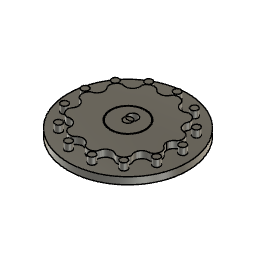
Example Result v0 (Autodesk Fusion 360 design; units mm, degrees)
Autodesk Fusion 360 part; units mm, degrees
sketch "diskSketch" plane through (0, 0, 0) normal (0, 0, 1) x (1, 0, 0)
  spline S0 degree 5 number of poles 1805
  spline S1 degree 5 number of poles 1805
  spline S2 degree 3 poles (27.5, 0) (27.5, -0.8364) (27.7298, -1.6288) (27.9895, -2.1783) (28.3571, -2.9563) (28.7204, -3.3302) (28.9647, -3.582) (29.3501, -3.9791) (29.5444, -4.104) (29.6826, -4.2063) (29.9351, -4.3932) (29.9974, -4.4285) (30.0646, -4.475) (30.2296, -4.589) (30.2633, -4.6167) (30.3364, -4.6819) (30.5367, -4.8606) (30.8163, -5.1989) (31.0395, -5.7169) (31.3799, -6.5067) (31.5244, -7.6667) (31.2804, -8.7782) (31.0439, -9.8558) (30.4517, -10.869) (29.7612, -11.5227) (29.2524, -12.0044) (28.7053, -12.2856) (28.3272, -12.3989) (28.1828, -12.4422) (28.0593, -12.4636) (27.9596, -12.4749) (27.9048, -12.4811) (27.8974, -12.4821) (27.7486, -12.4878) (27.6622, -12.4911) (27.5665, -12.4944) (27.4556, -12.4988) (27.3788, -12.5019) (27.2857, -12.4897) (26.842, -12.5475) (26.5223, -12.5891) (26.0046, -12.6545) (25.2479, -13.0138) (24.7458, -13.2522) (24.1194, -13.646) (23.5495, -14.3118) (23.0297, -14.919) (22.6138, -15.7656) (22.4459, -16.5212) (22.2613, -17.3526) (22.3204, -18.0094) (22.386, -18.4313) (22.4877, -19.0857) (22.5909, -19.29) (22.642, -19.4348) (22.7121, -19.6333) (22.7474, -19.717) (22.7899, -19.8212) (22.8708, -20.0199) (22.9081, -20.104) (22.9231, -20.142) (22.9596, -20.2349) (22.9966, -20.3483) (23.0229, -20.4798) (23.0861, -20.796) (23.1033, -21.3457) (22.941, -21.9659) (22.7031, -22.875) (22.0726, -23.9098) (21.187, -24.6432) (20.3584, -25.3292) (19.3241, -25.7421) (18.4538, -25.8362) (17.8604, -25.9004) (17.353, -25.8209) (17.045, -25.7203) (16.9404, -25.6861) (16.8631, -25.6529) (16.7756, -25.6098) (16.723, -25.584) (16.7225, -25.5844) (16.6515, -25.5425) (16.6091, -25.5175) (16.5151, -25.4606) (16.4071, -25.3973) (16.3212, -25.347) (16.2748, -25.3194) (16.1409, -25.2452) (16.052, -25.196) (15.9195, -25.1081) (15.5103, -24.9416) (15.1789, -24.8066) (14.6328, -24.6047) (13.8187, -24.5618) (13.0612, -24.5218) (12.0837, -24.6809) (11.2521, -25.0993) (10.3608, -25.5476) (9.6892, -26.2416) (9.296, -26.8297) (8.8257, -27.5333) (8.6839, -28.0536) (8.6021, -28.3468) (8.482, -28.7769) (8.489, -28.8266) (8.4745, -28.9021) (8.4406, -29.0782) (8.4026, -29.2946) (8.392, -29.3494) (8.3809, -29.4064) (8.3746, -29.4314) (8.3564, -29.4951) (8.316, -29.6367) (8.2697, -29.7576) (8.1789, -29.9291) (7.9347, -30.3903) (7.4012, -31.0102) (6.6342, -31.4665) (5.714, -32.014) (4.4821, -32.3033) (3.3558, -32.2059) (2.3425, -32.1183) (1.4347, -31.7209) (0.8897, -31.2936) (0.6133, -31.0769) (0.4328, -30.8653) (0.3291, -30.7121) (0.2863, -30.6489) (0.2436, -30.5766) (0.2081, -30.5089) (0.1823, -30.4595) (0.1408, -30.3648) (-0.0014, -30.0921) (-0.0541, -29.991) (-0.1025, -29.8918) (-0.2461, -29.6587) (-0.3423, -29.5025) (-0.4742, -29.2688) (-0.8391, -28.8643) (-1.1195, -28.5534) (-1.5694, -28.1164) (-2.2864, -27.7436) (-2.9439, -27.4017) (-3.8232, -27.1741) (-4.6043, -27.1692) (-5.4948, -27.1637) (-6.1979, -27.3848) (-6.6882, -27.5989) (-7.4716, -27.941) (-7.8317, -28.2711) (-8.0745, -28.4848) (-8.476, -28.8382) (-8.5172, -28.9164) (-8.5762, -28.9799) (-8.7072, -29.1206) (-8.8019, -29.2219) (-8.8412, -29.2609) (-8.912, -29.3312) (-9.005, -29.4114) (-9.1302, -29.4954) (-9.5088, -29.7495) (-10.2824, -30.0502) (-11.2002, -30.0607) (-12.294, -30.0733) (-13.5598, -29.6739) (-14.5105, -28.9669) (-15.3604, -28.3349) (-15.9413, -27.4715) (-16.1735, -26.797) (-16.2958, -26.442) (-16.3282, -26.1649) (-16.328, -25.9607) (-16.3279, -25.8747) (-16.3261, -25.8385) (-16.3063, -25.6536) (-16.2985, -25.5807) (-16.2912, -25.5258) (-16.2741, -25.3561) (-16.2616, -25.2314) (-16.2255, -25.0355) (-16.2432, -24.5221) (-16.2531, -24.2338) (-16.2694, -23.8438) (-16.4483, -23.2265) (-16.5847, -22.7558) (-16.8375, -22.1165) (-17.3604, -21.4595) (-17.8554, -20.8375) (-18.6109, -20.2666) (-19.3143, -19.9609) (-20.0832, -19.6267) (-20.7177, -19.5586) (-21.1477, -19.5403) (-21.8219, -19.5117) (-22.1004, -19.5816) (-22.307, -19.6171) (-22.6555, -19.6769) (-22.7856, -19.7171) (-22.8998, -19.7464) (-23.1587, -19.8128) (-23.1843, -19.8205) (-23.2501, -19.8343) (-23.4304, -19.8721) (-23.6097, -19.8913) (-23.8896, -19.8684) (-24.4796, -19.8201) (-25.3885, -19.5117) (-26.1748, -18.8757) (-27.0038, -18.2052) (-27.6841, -17.1908) (-27.9911, -16.1567) (-28.2675, -15.2257) (-28.235, -14.2921) (-28.0634, -13.6842) (-27.9892, -13.4213) (-27.9, -13.2271) (-27.815, -13.083) (-27.7771, -13.0188) (-27.7302, -12.9492) (-27.7028, -12.9124) (-27.6844, -12.8876) (-27.6489, -12.8431) (-27.5569, -12.7286) (-27.5038, -12.6625) (-27.4564, -12.6033) (-27.4033, -12.5363) (-27.3615, -12.4835) (-27.3087, -12.4318) (-27.1123, -12.1457) (-26.9522, -11.9125) (-26.6641, -11.5059) (-26.4205, -10.734) (-26.2398, -10.1613) (-26.1008, -9.3649) (-26.235, -8.4458) (-26.3558, -7.6193) (-26.739, -6.7287) (-27.2269, -6.0891) (-27.7439, -5.4112) (-28.294, -5.0252) (-28.665, -4.8012) (-29.2451, -4.451) (-29.4567, -4.4063) (-29.5843, -4.358) (-29.7507, -4.2949) (-29.8157, -4.2735) (-29.9166, -4.2392) (-30.0953, -4.1785) (-30.2009, -4.1453) (-30.2363, -4.133) (-30.2851, -4.116) (-30.3346, -4.0961) (-30.3964, -4.0682) (-30.5109, -4.0166) (-30.6072, -3.9633) (-30.742, -3.8694) (-31.1329, -3.5971) (-31.6402, -3.0544) (-31.9935, -2.3069) (-32.4399, -1.3624) (-32.6142, -0.118) (-32.4095, 1.0026) (-32.2576, 1.8342) (-31.9068, 2.5902) (-31.499, 3.1259) (-31.2419, 3.4636) (-30.9701, 3.711) (-30.7392, 3.8713) (-30.5825, 3.9801) (-30.4714, 4.0378) (-30.3366, 4.0942) (-30.2813, 4.1173) (-30.2756, 4.1201) (-30.1976, 4.1462) (-30.1459, 4.1634) (-30.0203, 4.2035) (-29.8763, 4.253) (-29.7877, 4.2834) (-29.728, 4.3034) (-29.5798, 4.3597) (-29.46, 4.4052) (-29.2683, 4.4545) (-28.7732, 4.7376) (-28.4321, 4.9327) (-27.9182, 5.2633) (-27.3929, 5.8827) (-26.9035, 6.4599) (-26.4683, 7.2978) (-26.293, 8.1223) (-26.0881, 9.0859) (-26.1992, 9.9611) (-26.3764, 10.5866) (-26.6142, 11.4261) (-26.925, 11.87) (-27.096, 12.1219) (-27.3408, 12.4823) (-27.3781, 12.5046) (-27.424, 12.5623) (-27.515, 12.6769) (-27.6332, 12.8228) (-27.6725, 12.8729) (-27.7163, 12.9287) (-27.7233, 12.9391) (-27.7575, 12.9911) (-27.8417, 13.1187) (-27.9123, 13.25) (-27.9871, 13.4502) (-28.1807, 13.9688) (-28.2892, 14.8359) (-28.0932, 15.7558) (-27.8673, 16.8165) (-27.2406, 17.9172) (-26.412, 18.672) (-25.665, 19.3525) (-24.769, 19.7379) (-24.1169, 19.841) (-23.7892, 19.8928) (-23.5487, 19.8831) (-23.3653, 19.8552) (-23.3028, 19.8457) (-23.2472, 19.8348) (-23.1696, 19.816) (-23.1079, 19.801) (-23.0329, 19.7773) (-22.7561, 19.7106) (-22.6382, 19.6821) (-22.5014, 19.6455) (-22.1939, 19.5988) (-21.9926, 19.5682) (-21.7155, 19.5183) (-21.1676, 19.5395) (-20.7578, 19.5554) (-20.1633, 19.6148) (-19.4304, 19.9121) (-18.7619, 20.1833) (-18.0201, 20.6943) (-17.5047, 21.2862) (-16.9391, 21.9357) (-16.6447, 22.6034) (-16.4874, 23.0977) (-16.2407, 23.8734) (-16.2454, 24.3147) (-16.2406, 24.6279) (-16.232, 25.1873) (-16.2715, 25.3348) (-16.2831, 25.442) (-16.3005, 25.6029) (-16.3098, 25.6825) (-16.3165, 25.753) (-16.3288, 25.8813) (-16.3292, 25.9161) (-16.3276, 26.0013) (-16.3228, 26.2464) (-16.2669, 26.5994) (-16.0832, 27.0318) (-15.7711, 27.7665) (-15.0765, 28.6349) (-14.1404, 29.2194) (-13.1966, 29.8087) (-12.0276, 30.1013) (-11.0333, 30.056) (-10.3394, 30.0243) (-9.7408, 29.8356) (-9.3544, 29.6294) (-9.1559, 29.5235) (-9.0203, 29.4228) (-8.912, 29.3271) (-8.8658, 29.2862) (-8.8531, 29.2748) (-8.7838, 29.202) (-8.7349, 29.1507) (-8.6604, 29.0703) (-8.5751, 28.9786) (-8.5254, 28.9252) (-8.4787, 28.8629) (-8.2345, 28.6311) (-8.049, 28.4551) (-7.7634, 28.1655) (-7.1134, 27.8081) (-6.7184, 27.5909) (-6.1661, 27.3374) (-5.3667, 27.2217) (-4.6642, 27.1201) (-3.7569, 27.1776) (-2.9737, 27.4481) (-2.162, 27.7285) (-1.5452, 28.1805) (-1.1609, 28.5377) (-0.598, 29.0607) (-0.4197, 29.3848) (-0.2935, 29.5829) (-0.1127, 29.8668) (-0.066, 29.9688) (-0.0091, 30.0774) (0.2217, 30.5179) (0.2057, 30.5088) (0.2538, 30.5917) (0.3361, 30.7335) (0.4253, 30.8582) (0.5862, 31.0229) (0.9753, 31.4213) (1.7542, 31.9081) (2.7129, 32.1108) (3.7766, 32.3358) (5.0356, 32.2101) (6.0583, 31.7621) (6.7284, 31.4686) (7.2951, 31.0465) (7.6822, 30.6225) (7.9524, 30.3264) (8.1342, 30.0354) (8.243, 29.7997) (8.3005, 29.6752) (8.3306, 29.5884) (8.3609, 29.4793) (8.3778, 29.4183) (8.3814, 29.4047) (8.3938, 29.3399) (8.403, 29.2915) (8.4292, 29.1419) (8.455, 29.0044) (8.47, 28.9245) (8.474, 28.8947) (8.5108, 28.721) (8.5373, 28.5959) (8.5681, 28.3644) (8.7663, 27.8511) (8.9305, 27.426) (9.2319, 26.7809) (9.8645, 26.1231) (10.415, 25.5505) (11.2404, 25.0128) (12.1257, 24.7564) (13.026, 24.4956) (13.9153, 24.5301) (14.5283, 24.6489) (15.3068, 24.7998) (15.6828, 25.01) (15.8931, 25.1147) (16.1845, 25.2599) (16.2151, 25.2865) (16.285, 25.3266) (16.4234, 25.406) (16.5925, 25.5077) (16.6517, 25.5426) (16.7242, 25.5854) (16.7249, 25.5851) (16.7795, 25.6118) (16.9246, 25.6828) (17.0645, 25.7361) (17.2801, 25.7845) (17.7791, 25.8965) (18.5768, 25.8984) (19.4027, 25.631) (20.4105, 25.3047) (21.4331, 24.5804) (22.1043, 23.6778) (22.6277, 22.9741) (22.9366, 22.1737) (23.0328, 21.5172) (23.1018, 21.0463) (23.0627, 20.6449) (23.0093, 20.4173) (22.9887, 20.3292) (22.9554, 20.2264) (22.93, 20.1597) (22.9153, 20.1214) (22.8933, 20.0721) (22.8111, 19.873) (22.7704, 19.7744) (22.7302, 19.6763) (22.672, 19.518) (22.6324, 19.4102) (22.572, 19.2776) (22.4727, 18.8679) (22.3989, 18.5631) (22.2832, 18.0707) (22.3357, 17.2884) (22.3779, 16.6599) (22.5777, 15.8389) (22.9826, 15.1214) (23.4111, 14.362) (24.0166, 13.779) (24.5504, 13.4143) (25.3758, 12.8504) (26.0286, 12.6983) (26.4611, 12.6107) (27.123, 12.4766) (27.3047, 12.5052) (27.4079, 12.5008) (27.5295, 12.4956) (27.5867, 12.4938) (27.6726, 12.4906) (27.8267, 12.4849) (27.8822, 12.4822) (27.9215, 12.4787) (27.9981, 12.472) (28.125, 12.4535) (28.2503, 12.4206) (28.6521, 12.315) (29.3279, 11.9787) (29.9133, 11.372) (30.6239, 10.6357) (31.1877, 9.5184) (31.3523, 8.383) (31.5133, 7.2733) (31.2858, 6.169) (30.9215, 5.4678) (30.7394, 5.1172) (30.5374, 4.8717) (30.3815, 4.7234) (30.3035, 4.6493) (30.2602, 4.6127) (30.1351, 4.5242) (30.0815, 4.4862) (30.0264, 4.4499) (29.8663, 4.3382) (29.7692, 4.2704) (29.6334, 4.1879) (29.3172, 3.9145) (29.1277, 3.7506) (28.8612, 3.5354) (28.4682, 2.9898) (28.2075, 2.6278) (27.8772, 2.0856) (27.67, 1.3043) (27.565, 0.9081) (27.5, 0.4556) (27.5, 0) knots 0 0 0 0 0.0004895 0.0004895 0.0004895 0.00118259 0.00118259 0.00118259 0.00227595 0.00227595 0.00227595 0.00427422 0.00427422 0.00427422 0.00917873 0.00917873 0.00917873 0.02262065 0.02262065 0.02262065 0.04311537 0.04311537 0.04311537 0.0629846 0.0629846 0.0629846 0.07762546 0.07762546 0.07762546 0.08321474 0.08321474 0.08321474 0.08628579 0.08628579 0.08628579 0.08807039 0.08807039 0.08807039 0.08930494 0.08930494 0.08930494 0.09019429 0.09019429 0.09019429 0.09078445 0.09078445 0.09078445 0.09132266 0.09132266 0.09132266 0.09191484 0.09191484 0.09191484 0.09283321 0.09283321 0.09283321 0.09409235 0.09409235 0.09409235 0.09649245 0.09649245 0.09649245 0.10235615 0.10235615 0.10235615 0.11645429 0.11645429 0.11645429 0.13711768 0.13711768 0.13711768 0.15644901 0.15644901 0.15644901 0.1696295 0.1696295 0.1696295 0.1741071 0.1741071 0.1741071 0.17679588 0.17679588 0.17679588 0.1784037 0.1784037 0.1784037 0.17968093 0.17968093 0.17968093 0.18052857 0.18052857 0.18052857 0.18121516 0.18121516 0.18121516 0.18185402 0.18185402 0.18185402 0.18253869 0.18253869 0.18253869 0.18335769 0.18335769 0.18335769 0.18455897 0.18455897 0.18455897 0.18735939 0.18735939 0.18735939 0.19026496 0.19026496 0.19026496 0.19672698 0.19672698 0.19672698 0.21410686 0.21410686 0.21410686 0.2349604 0.2349604 0.2349604 0.25372072 0.25372072 0.25372072 0.26323468 0.26323468 0.26323468 0.26716265 0.26716265 0.26716265 0.2700253 0.2700253 0.2700253 0.27108749 0.27108749 0.27108749 0.27179932 0.27179932 0.27179932 0.27234648 0.27234648 0.27234648 0.27284827 0.27284827 0.27284827 0.2734204 0.2734204 0.2734204 0.27433454 0.27433454 0.27433454 0.27584592 0.27584592 0.27584592 0.27920032 0.27920032 0.27920032 0.28524135 0.28524135 0.28524135 0.30350219 0.30350219 0.30350219 0.32526775 0.32526775 0.32526775 0.344725 0.344725 0.344725 0.35496367 0.35496367 0.35496367 0.35927589 0.35927589 0.35927589 0.36097586 0.36097586 0.36097586 0.36222396 0.36222396 0.36222396 0.36292478 0.36292478 0.36292478 0.36345931 0.36345931 0.36345931 0.36396532 0.36396532 0.36396532 0.36451839 0.36451839 0.36451839 0.3653857 0.3653857 0.3653857 0.36684904 0.36684904 0.36684904 0.37016576 0.37016576 0.37016576 0.37924482 0.37924482 0.37924482 0.39838777 0.39838777 0.39838777 0.41856891 0.41856891 0.41856891 0.43673863 0.43673863 0.43673863 0.44459901 0.44459901 0.44459901 0.44809961 0.44809961 0.44809961 0.4504535 0.4504535 0.4504535 0.45181271 0.45181271 0.45181271 0.45288339 0.45288339 0.45288339 0.45375646 0.45375646 0.45375646 0.4544043 0.4544043 0.4544043 0.45498694 0.45498694 0.45498694 0.45560434 0.45560434 0.45560434 0.45656983 0.45656983 0.45656983 0.45782948 0.45782948 0.45782948 0.46005992 0.46005992 0.46005992 0.46312902 0.46312902 0.46312902 0.46880455 0.46880455 0.46880455 0.48526725 0.48526725 0.48526725 0.5060698 0.5060698 0.5060698 0.52150512 0.52150512 0.52150512 0.53123486 0.53123486 0.53123486 0.53783732 0.53783732 0.53783732 0.54054314 0.54054314 0.54054314 0.54233789 0.54233789 0.54233789 0.5434415 0.5434415 0.5434415 0.54433321 0.54433321 0.54433321 0.54494776 0.54494776 0.54494776 0.54552032 0.54552032 0.54552032 0.54618951 0.54618951 0.54618951 0.54708756 0.54708756 0.54708756 0.54837287 0.54837287 0.54837287 0.55092383 0.55092383 0.55092383 0.55376597 0.55376597 0.55376597 0.56074285 0.56074285 0.56074285 0.57881743 0.57881743 0.57881743 0.59965766 0.59965766 0.59965766 0.61844581 0.61844581 0.61844581 0.62788938 0.62788938 0.62788938 0.63111017 0.63111017 0.63111017 0.63366994 0.63366994 0.63366994 0.63475964 0.63475964 0.63475964 0.635473 0.635473 0.635473 0.63600667 0.63600667 0.63600667 0.63649349 0.63649349 0.63649349 0.63702765 0.63702765 0.63702765 0.63786593 0.63786593 0.63786593 0.63936372 0.63936372 0.63936372 0.64160996 0.64160996 0.64160996 0.64569763 0.64569763 0.64569763 0.65746357 0.65746357 0.65746357 0.67745587 0.67745587 0.67745587 0.69761487 0.69761487 0.69761487 0.7116825 0.7116825 0.7116825 0.71890829 0.71890829 0.71890829 0.72199175 0.72199175 0.72199175 0.72416369 0.72416369 0.72416369 0.72543114 0.72543114 0.72543114 0.72639376 0.72639376 0.72639376 0.72697867 0.72697867 0.72697867 0.72749264 0.72749264 0.72749264 0.72802538 0.72802538 0.72802538 0.7288056 0.7288056 0.7288056 0.72992363 0.72992363 0.72992363 0.73445822 0.73445822 0.73445822 0.74221478 0.74221478 0.74221478 0.76097264 0.76097264 0.76097264 0.78178556 0.78178556 0.78178556 0.79542396 0.79542396 0.79542396 0.80494586 0.80494586 0.80494586 0.80997549 0.80997549 0.80997549 0.81279025 0.81279025 0.81279025 0.81489378 0.81489378 0.81489378 0.81611582 0.81611582 0.81611582 0.81699629 0.81699629 0.81699629 0.81772554 0.81772554 0.81772554 0.81836023 0.81836023 0.81836023 0.81900578 0.81900578 0.81900578 0.81982558 0.81982558 0.81982558 0.82096133 0.82096133 0.82096133 0.8232058 0.8232058 0.8232058 0.8259593 0.8259593 0.8259593 0.83328439 0.83328439 0.83328439 0.85024081 0.85024081 0.85024081 0.87093352 0.87093352 0.87093352 0.88706683 0.88706683 0.88706683 0.89863825 0.89863825 0.89863825 0.90311813 0.90311813 0.90311813 0.9056923 0.9056923 0.9056923 0.90696765 0.90696765 0.90696765 0.90783657 0.90783657 0.90783657 0.90848293 0.90848293 0.90848293 0.90900219 0.90900219 0.90900219 0.90955175 0.90955175 0.90955175 0.9104014 0.9104014 0.9104014 0.91170187 0.91170187 0.91170187 0.91323489 0.91323489 0.91323489 0.91598534 0.91598534 0.91598534 0.92133468 0.92133468 0.92133468 0.9384865 0.9384865 0.9384865 0.95930437 0.95930437 0.95930437 0.97965218 0.97965218 0.97965218 0.98982609 0.98982609 0.98982609 0.99491305 0.99491305 0.99491305 0.99709279 0.99709279 0.99709279 0.99841498 0.99841498 0.99841498 0.99920749 0.99920749 0.99920749 0.99973334 0.99973334 0.99973334 1 1 1 1
  circle A0 centre (0, 0) radius 12.5
  point P0 (32.5492, -0.096)
  point P1 (32.6945, -0.2144)
  point P2 (32.9288, -0.3765)
  point P3 (33.2407, -0.6017)
  point P4 (33.615, -0.9067)
  point P5 (34.0333, -1.3046)
  point P6 (34.4748, -1.8043)
  point P7 (34.9171, -2.4105)
  point P8 (35.3377, -3.123)
  point P9 (35.7141, -3.9367)
  point P10 (36.0256, -4.8423)
  point P11 (36.2537, -5.8263)
  point P12 (36.3833, -6.8717)
  point P13 (36.403, -7.9585)
  point P14 (36.3057, -9.0651)
  point P15 (36.089, -10.1688)
  point P16 (35.7555, -11.2468)
  point P17 (35.312, -12.2774)
  point P18 (34.7701, -13.2409)
  point P19 (34.145, -14.1201)
  point P20 (33.4551, -14.9017)
  point P21 (32.7214, -15.5763)
  point P22 (31.9661, -16.139)
  point P23 (31.2121, -16.5898)
  point P24 (30.4818, -16.9332)
  point P25 (29.796, -17.1783)
  point P26 (29.1733, -17.3384)
  point P27 (28.629, -17.4302)
  point P28 (28.1747, -17.4731)
  point P29 (27.8174, -17.4887)
  point P30 (27.5599, -17.4993)
  point P31 (27.3998, -17.5272)
  point P32 (27.3302, -17.5941)
  point P33 (27.34, -17.7191)
  point P34 (27.414, -17.9192)
  point P35 (27.534, -18.2073)
  point P36 (27.6794, -18.5925)
  point P37 (27.8281, -19.0793)
  point P38 (27.9574, -19.6675)
  point P39 (28.0451, -20.3522)
  point P40 (28.0706, -21.1239)
  point P41 (28.0156, -21.9691)
  point P42 (27.865, -22.8706)
  point P43 (27.6073, -23.8088)
  point P44 (27.2358, -24.7617)
  point P45 (26.748, -25.7068)
  point P46 (26.1464, -26.6211)
  point P47 (25.4381, -27.4831)
  point P48 (24.6346, -28.273)
  point P49 (23.751, -28.9737)
  point P50 (22.806, -29.5719)
  point P51 (21.8203, -30.0582)
  point P52 (20.8164, -30.4279)
  point P53 (19.817, -30.6809)
  point P54 (18.8445, -30.8219)
  point P55 (17.9199, -30.8601)
  point P56 (17.0617, -30.8088)
  point P57 (16.2852, -30.6849)
  point P58 (15.6021, -30.508)
  point P59 (15.0196, -30.2996)
  point P60 (14.5402, -30.0824)
  point P61 (14.1619, -29.8788)
  point P62 (13.8777, -29.7104)
  point P63 (13.6766, -29.5968)
  point P64 (13.5437, -29.5547)
  point P65 (13.4607, -29.5976)
  point P66 (13.4072, -29.7344)
  point P67 (13.3612, -29.9697)
  point P68 (13.3001, -30.3036)
  point P69 (13.2019, -30.7311)
  point P70 (13.0461, -31.2428)
  point P71 (12.8146, -31.8252)
  point P72 (12.4922, -32.4615)
  point P73 (12.0677, -33.1316)
  point P74 (11.5344, -33.814)
  point P75 (10.89, -34.4858)
  point P76 (10.137, -35.1245)
  point P77 (9.2825, -35.7083)
  point P78 (8.338, -36.2174)
  point P79 (7.319, -36.6349)
  point P80 (6.2437, -36.9474)
  point P81 (5.1333, -37.1456)
  point P82 (4.0099, -37.2247)
  point P83 (2.8964, -37.1848)
  point P84 (1.8153, -37.0306)
  point P85 (0.7873, -36.7713)
  point P86 (-0.169, -36.4204)
  point P87 (-1.0383, -35.9947)
  point P88 (-1.809, -35.5141)
  point P89 (-2.474, -35.0001)
  point P90 (-3.0306, -34.4754)
  point P91 (-3.4812, -33.9627)
  point P92 (-3.8324, -33.4838)
  point P93 (-4.0956, -33.0582)
  point P94 (-4.2855, -32.7031)
  point P95 (-4.4205, -32.4317)
  point P96 (-4.5209, -32.2535)
  point P97 (-4.6088, -32.1732)
  point P98 (-4.7067, -32.1908)
  point P99 (-4.8365, -32.3017)
  point P100 (-5.0187, -32.4965)
  point P101 (-5.2715, -32.7621)
  point P102 (-5.6098, -33.0815)
  point P103 (-6.0447, -33.4349)
  point P104 (-6.583, -33.8009)
  point P105 (-7.2269, -34.1568)
  point P106 (-7.9739, -34.48)
  point P107 (-8.8166, -34.7489)
  point P108 (-9.7436, -34.9437)
  point P109 (-10.7394, -35.0475)
  point P110 (-11.7856, -35.0471)
  point P111 (-12.8612, -34.9332)
  point P112 (-13.9439, -34.701)
  point P113 (-15.0108, -34.3506)
  point P114 (-16.0396, -33.8868)
  point P115 (-17.0094, -33.3188)
  point P116 (-17.9017, -32.66)
  point P117 (-18.7013, -31.9275)
  point P118 (-19.3966, -31.141)
  point P119 (-19.9805, -30.3222)
  point P120 (-20.4507, -29.4938)
  point P121 (-20.8092, -28.6786)
  point P122 (-21.0631, -27.8982)
  point P123 (-21.2236, -27.1727)
  point P124 (-21.3058, -26.5189)
  point P125 (-21.328, -25.9504)
  point P126 (-21.3106, -25.4767)
  point P127 (-21.2759, -25.1026)
  point P128 (-21.2464, -24.8284)
  point P129 (-21.2441, -24.6494)
  point P130 (-21.2896, -24.5567)
  point P131 (-21.4011, -24.537)
  point P132 (-21.5936, -24.5736)
  point P133 (-21.8782, -24.647)
  point P134 (-22.2618, -24.7357)
  point P135 (-22.7466, -24.8173)
  point P136 (-23.3299, -24.8693)
  point P137 (-24.0046, -24.8701)
  point P138 (-24.7591, -24.8003)
  point P139 (-25.5781, -24.643)
  point P140 (-26.4429, -24.385)
  point P141 (-27.3327, -24.0171)
  point P142 (-28.225, -23.5347)
  point P143 (-29.0971, -22.9378)
  point P144 (-29.9266, -22.2313)
  point P145 (-30.6927, -21.4244)
  point P146 (-31.3768, -20.5307)
  point P147 (-31.9636, -19.5671)
  point P148 (-32.4419, -18.5533)
  point P149 (-32.8044, -17.5112)
  point P150 (-33.0488, -16.4635)
  point P151 (-33.1775, -15.4327)
  point P152 (-33.1973, -14.4409)
  point P153 (-33.1197, -13.5076)
  point P154 (-32.9599, -12.6501)
  point P155 (-32.7362, -11.8818)
  point P156 (-32.4693, -11.2123)
  point P157 (-32.1815, -10.6463)
  point P158 (-31.8955, -10.1842)
  point P159 (-31.6335, -9.8214)
  point P160 (-31.4162, -9.549)
  point P161 (-31.2619, -9.3538)
  point P162 (-31.1859, -9.2192)
  point P163 (-31.1993, -9.1258)
  point P164 (-31.3092, -9.0521)
  point P165 (-31.5178, -8.9759)
  point P166 (-31.8227, -8.8748)
  point P167 (-32.2167, -8.7274)
  point P168 (-32.6884, -8.5142)
  point P169 (-33.2226, -8.2186)
  point P170 (-33.8006, -7.8274)
  point P171 (-34.4017, -7.3316)
  point P172 (-35.0036, -6.7266)
  point P173 (-35.5833, -6.0125)
  point P174 (-36.1187, -5.1943)
  point P175 (-36.5889, -4.2814)
  point P176 (-36.9753, -3.2871)
  point P177 (-37.2629, -2.2286)
  point P178 (-37.4401, -1.1257)
  point P179 (-37.5, 0)
  point P180 (-37.4401, 1.1257)
  point P181 (-37.2629, 2.2286)
  point P182 (-36.9753, 3.2871)
  point P183 (-36.5889, 4.2814)
  point P184 (-36.1187, 5.1943)
  point P185 (-35.5833, 6.0125)
  point P186 (-35.0036, 6.7266)
  point P187 (-34.4017, 7.3316)
  point P188 (-33.8006, 7.8274)
  point P189 (-33.2226, 8.2186)
  point P190 (-32.6884, 8.5142)
  point P191 (-32.2167, 8.7274)
  point P192 (-31.8227, 8.8748)
  point P193 (-31.5178, 8.9759)
  point P194 (-31.3092, 9.0521)
  point P195 (-31.1993, 9.1258)
  point P196 (-31.1859, 9.2192)
  point P197 (-31.2619, 9.3538)
  point P198 (-31.4162, 9.549)
  point P199 (-31.6335, 9.8214)
  point P200 (-31.8955, 10.1842)
  point P201 (-32.1815, 10.6463)
  point P202 (-32.4693, 11.2123)
  point P203 (-32.7362, 11.8818)
  point P204 (-32.9599, 12.6501)
  point P205 (-33.1197, 13.5076)
  point P206 (-33.1973, 14.4409)
  point P207 (-33.1775, 15.4327)
  point P208 (-33.0488, 16.4635)
  point P209 (-32.8044, 17.5112)
  point P210 (-32.4419, 18.5533)
  point P211 (-31.9636, 19.5671)
  point P212 (-31.3768, 20.5307)
  point P213 (-30.6927, 21.4244)
  point P214 (-29.9266, 22.2313)
  point P215 (-29.0971, 22.9378)
  point P216 (-28.225, 23.5347)
  point P217 (-27.3327, 24.0171)
  point P218 (-26.4429, 24.385)
  point P219 (-25.5781, 24.643)
  point P220 (-24.7591, 24.8003)
  point P221 (-24.0046, 24.8701)
  point P222 (-23.3299, 24.8693)
  point P223 (-22.7466, 24.8173)
  point P224 (-22.2618, 24.7357)
  point P225 (-21.8782, 24.647)
  point P226 (-21.5936, 24.5736)
  point P227 (-21.4011, 24.537)
  point P228 (-21.2896, 24.5567)
  point P229 (-21.2441, 24.6494)
  point P230 (-21.2464, 24.8284)
  point P231 (-21.2759, 25.1026)
  point P232 (-21.3106, 25.4767)
  point P233 (-21.328, 25.9504)
  point P234 (-21.3058, 26.5189)
  point P235 (-21.2236, 27.1727)
  point P236 (-21.0631, 27.8982)
  point P237 (-20.8092, 28.6786)
  point P238 (-20.4507, 29.4938)
  point P239 (-19.9805, 30.3222)
  point P240 (-19.3966, 31.141)
  point P241 (-18.7013, 31.9275)
  point P242 (-17.9017, 32.66)
  point P243 (-17.0094, 33.3188)
  point P244 (-16.0396, 33.8868)
  point P245 (-15.0108, 34.3506)
  point P246 (-13.9439, 34.701)
  point P247 (-12.8612, 34.9332)
  point P248 (-11.7856, 35.0471)
  point P249 (-10.7394, 35.0475)
  point P250 (-9.7436, 34.9437)
  point P251 (-8.8166, 34.7489)
  point P252 (-7.9739, 34.48)
  point P253 (-7.2269, 34.1568)
  point P254 (-6.583, 33.8009)
  point P255 (-6.0447, 33.4349)
  point P256 (-5.6098, 33.0815)
  point P257 (-5.2715, 32.7621)
  point P258 (-5.0187, 32.4965)
  point P259 (-4.8365, 32.3017)
  point P260 (-4.7067, 32.1908)
  point P261 (-4.6088, 32.1732)
  point P262 (-4.5209, 32.2535)
  point P263 (-4.2855, 32.7031)
  point P264 (-4.0956, 33.0582)
  point P265 (-3.8324, 33.4838)
  point P266 (-3.4812, 33.9627)
  point P267 (-3.0306, 34.4754)
  point P268 (-2.474, 35.0001)
  point P269 (-1.809, 35.5141)
  point P270 (-1.0383, 35.9947)
  point P271 (-0.169, 36.4204)
  point P272 (0.7873, 36.7713)
  point P273 (1.8153, 37.0306)
  point P274 (2.8964, 37.1848)
  point P275 (4.0099, 37.2247)
  point P276 (5.1333, 37.1456)
  point P277 (6.2437, 36.9474)
  point P278 (7.319, 36.6349)
  point P279 (8.338, 36.2174)
  point P280 (9.2825, 35.7083)
  point P281 (10.137, 35.1245)
  point P282 (10.89, 34.4858)
  point P283 (11.5344, 33.814)
  point P284 (12.0677, 33.1316)
  point P285 (12.4922, 32.4615)
  point P286 (12.8146, 31.8252)
  point P287 (13.0461, 31.2428)
  point P288 (13.2019, 30.7311)
  point P289 (13.3001, 30.3036)
  point P290 (13.3612, 29.9697)
  point P291 (13.4072, 29.7344)
  point P292 (13.4607, 29.5976)
  point P293 (13.5437, 29.5547)
  point P294 (13.6766, 29.5968)
  point P295 (13.8777, 29.7104)
  point P296 (14.1619, 29.8788)
  point P297 (14.5402, 30.0824)
  point P298 (15.0196, 30.2996)
  point P299 (15.6021, 30.508)
  point P300 (16.2852, 30.6849)
  point P301 (17.0617, 30.8088)
  point P302 (17.9199, 30.8601)
  point P303 (18.8445, 30.8219)
  point P304 (19.817, 30.6809)
  point P305 (20.8164, 30.4279)
  point P306 (21.8203, 30.0582)
  point P307 (22.806, 29.5719)
  point P308 (23.751, 28.9737)
  point P309 (24.6346, 28.273)
  point P310 (25.4381, 27.4831)
  point P311 (26.1464, 26.6211)
  point P312 (26.748, 25.7068)
  point P313 (27.2358, 24.7617)
  point P314 (27.6073, 23.8088)
  point P315 (27.865, 22.8706)
  point P316 (28.0156, 21.9691)
  point P317 (28.0706, 21.1239)
  point P318 (28.0451, 20.3522)
  point P319 (27.9574, 19.6675)
  point P320 (27.8281, 19.0793)
  point P321 (27.6794, 18.5925)
  point P322 (27.534, 18.2073)
  point P323 (27.414, 17.9192)
  point P324 (27.34, 17.7191)
  point P325 (27.3302, 17.5941)
  point P326 (27.3998, 17.5272)
  point P327 (27.5599, 17.4993)
  point P328 (27.8174, 17.4887)
  point P329 (28.1747, 17.4731)
  point P330 (28.629, 17.4302)
  point P331 (29.1733, 17.3384)
  point P332 (29.796, 17.1783)
  point P333 (30.4818, 16.9332)
  point P334 (31.2121, 16.5898)
  point P335 (31.9661, 16.139)
  point P336 (32.7214, 15.5763)
  point P337 (33.4551, 14.9017)
  point P338 (34.145, 14.1201)
  point P339 (34.7701, 13.2409)
  point P340 (35.312, 12.2774)
  point P341 (35.7555, 11.2468)
  point P342 (36.089, 10.1688)
  point P343 (36.3057, 9.0651)
  point P344 (36.403, 7.9585)
  point P345 (36.3833, 6.8717)
  point P346 (36.2537, 5.8263)
  point P347 (36.0256, 4.8423)
  point P348 (35.7141, 3.9367)
  point P349 (35.3377, 3.123)
  point P350 (34.9171, 2.4105)
  point P351 (34.4748, 1.8043)
  point P352 (34.0333, 1.3046)
  point P353 (33.615, 0.9067)
  point P354 (33.2407, 0.6017)
  point P355 (32.9288, 0.3765)
  point P356 (32.6945, 0.2144)
  point P357 (32.5492, 0.096)
  point P358 (32.5492, -0.096)
  point P359 (32.6945, -0.2144)
  point P360 (32.9288, -0.3765)
  point P361 (33.2407, -0.6017)
  point P362 (33.615, -0.9067)
  point P363 (34.0333, -1.3046)
  point P364 (34.4748, -1.8043)
  point P365 (34.9171, -2.4105)
  point P366 (35.3377, -3.123)
  point P367 (35.7141, -3.9367)
  point P368 (36.0256, -4.8423)
  point P369 (36.2537, -5.8263)
  point P370 (36.3833, -6.8717)
  point P371 (36.403, -7.9585)
  point P372 (36.3057, -9.0651)
  point P373 (36.089, -10.1688)
  point P374 (35.7555, -11.2468)
  point P375 (35.312, -12.2774)
  point P376 (34.7701, -13.2409)
  point P377 (34.145, -14.1201)
  point P378 (33.4551, -14.9017)
  point P379 (32.7214, -15.5763)
  point P380 (31.9661, -16.139)
  point P381 (31.2121, -16.5898)
  point P382 (30.4818, -16.9332)
  point P383 (29.796, -17.1783)
  point P384 (29.1733, -17.3384)
  point P385 (28.629, -17.4302)
  point P386 (28.1747, -17.4731)
  point P387 (27.8174, -17.4887)
  point P388 (27.5599, -17.4993)
  point P389 (27.3998, -17.5272)
  point P390 (27.3302, -17.5941)
  point P391 (27.34, -17.7191)
  point P392 (27.414, -17.9192)
  point P393 (27.534, -18.2073)
  point P394 (27.6794, -18.5925)
  point P395 (27.8281, -19.0793)
  point P396 (27.9574, -19.6675)
  point P397 (28.0451, -20.3522)
  point P398 (28.0706, -21.1239)
  point P399 (28.0156, -21.9691)
  point P400 (27.865, -22.8706)
  point P401 (27.6073, -23.8088)
  point P402 (27.2358, -24.7617)
  point P403 (26.748, -25.7068)
  point P404 (26.1464, -26.6211)
  point P405 (25.4381, -27.4831)
  point P406 (24.6346, -28.273)
  point P407 (23.751, -28.9737)
  point P408 (22.806, -29.5719)
  point P409 (21.8203, -30.0582)
  point P410 (20.8164, -30.4279)
  point P411 (19.817, -30.6809)
  point P412 (18.8445, -30.8219)
  point P413 (17.9199, -30.8601)
  point P414 (17.0617, -30.8088)
  point P415 (16.2852, -30.6849)
  point P416 (15.6021, -30.508)
  point P417 (15.0196, -30.2996)
  point P418 (14.5402, -30.0824)
  point P419 (14.1619, -29.8788)
  point P420 (13.8777, -29.7104)
  point P421 (13.6766, -29.5968)
  point P422 (13.5437, -29.5547)
  point P423 (13.4607, -29.5976)
  point P424 (13.4072, -29.7344)
  point P425 (13.3612, -29.9697)
  point P426 (13.3001, -30.3036)
  point P427 (13.2019, -30.7311)
  point P428 (13.0461, -31.2428)
  point P429 (12.8146, -31.8252)
  point P430 (12.4922, -32.4615)
  point P431 (12.0677, -33.1316)
  point P432 (11.5344, -33.814)
  point P433 (10.89, -34.4858)
  point P434 (10.137, -35.1245)
  point P435 (9.2825, -35.7083)
  point P436 (8.338, -36.2174)
  point P437 (7.319, -36.6349)
  point P438 (6.2437, -36.9474)
  point P439 (5.1333, -37.1456)
  point P440 (4.0099, -37.2247)
  point P441 (2.8964, -37.1848)
  point P442 (1.8153, -37.0306)
  point P443 (0.7873, -36.7713)
  point P444 (-0.169, -36.4204)
  point P445 (-1.0383, -35.9947)
  point P446 (-1.809, -35.5141)
  point P447 (-2.474, -35.0001)
  point P448 (-3.0306, -34.4754)
  point P449 (-3.4812, -33.9627)
  point P450 (-3.8324, -33.4838)
  point P451 (-4.0956, -33.0582)
  point P452 (-4.2855, -32.7031)
  point P453 (-4.4205, -32.4317)
  point P454 (-4.5209, -32.2535)
  point P455 (-4.6088, -32.1732)
  point P456 (-4.7067, -32.1908)
  point P457 (-4.8365, -32.3017)
  point P458 (-5.0187, -32.4965)
  point P459 (-5.2715, -32.7621)
  point P460 (-5.6098, -33.0815)
  point P461 (-6.0447, -33.4349)
  point P462 (-6.583, -33.8009)
  point P463 (-7.2269, -34.1568)
  point P464 (-7.9739, -34.48)
  point P465 (-8.8166, -34.7489)
  point P466 (-9.7436, -34.9437)
  point P467 (-10.7394, -35.0475)
  point P468 (-11.7856, -35.0471)
  point P469 (-12.8612, -34.9332)
  point P470 (-13.9439, -34.701)
  point P471 (-15.0108, -34.3506)
  point P472 (-16.0396, -33.8868)
  point P473 (-17.0094, -33.3188)
  point P474 (-17.9017, -32.66)
  point P475 (-18.7013, -31.9275)
  point P476 (-19.3966, -31.141)
  point P477 (-19.9805, -30.3222)
  point P478 (-20.4507, -29.4938)
  point P479 (-20.8092, -28.6786)
  point P480 (-21.0631, -27.8982)
  point P481 (-21.2236, -27.1727)
  point P482 (-21.3058, -26.5189)
  point P483 (-21.328, -25.9504)
  point P484 (-21.3106, -25.4767)
  point P485 (-21.2759, -25.1026)
  point P486 (-21.2464, -24.8284)
  point P487 (-21.2441, -24.6494)
  point P488 (-21.2896, -24.5567)
  point P489 (-21.4011, -24.537)
  point P490 (-21.5936, -24.5736)
  point P491 (-21.8782, -24.647)
  point P492 (-22.2618, -24.7357)
  point P493 (-22.7466, -24.8173)
  point P494 (-23.3299, -24.8693)
  point P495 (-24.0046, -24.8701)
  point P496 (-24.7591, -24.8003)
  point P497 (-25.5781, -24.643)
  point P498 (-26.4429, -24.385)
  point P499 (-27.3327, -24.0171)
  point P500 (-28.225, -23.5347)
  point P501 (-29.0971, -22.9378)
  point P502 (-29.9266, -22.2313)
  point P503 (-30.6927, -21.4244)
  point P504 (-31.3768, -20.5307)
  point P505 (-31.9636, -19.5671)
  point P506 (-32.4419, -18.5533)
  point P507 (-32.8044, -17.5112)
  point P508 (-33.0488, -16.4635)
  point P509 (-33.1775, -15.4327)
  point P510 (-33.1973, -14.4409)
  point P511 (-33.1197, -13.5076)
  point P512 (-32.9599, -12.6501)
  point P513 (-32.7362, -11.8818)
  point P514 (-32.4693, -11.2123)
  point P515 (-32.1815, -10.6463)
  point P516 (-31.8955, -10.1842)
  point P517 (-31.6335, -9.8214)
  point P518 (-31.4162, -9.549)
  point P519 (-31.2619, -9.3538)
  point P520 (-31.1859, -9.2192)
  point P521 (-31.1993, -9.1258)
  point P522 (-31.3092, -9.0521)
  point P523 (-31.5178, -8.9759)
  point P524 (-31.8227, -8.8748)
  point P525 (-32.2167, -8.7274)
  point P526 (-32.6884, -8.5142)
  point P527 (-33.2226, -8.2186)
  point P528 (-33.8006, -7.8274)
  point P529 (-34.4017, -7.3316)
  point P530 (-35.0036, -6.7266)
  point P531 (-35.5833, -6.0125)
  point P532 (-36.1187, -5.1943)
  point P533 (-36.5889, -4.2814)
  point P534 (-36.9753, -3.2871)
  point P535 (-37.2629, -2.2286)
  point P536 (-37.4401, -1.1257)
  point P537 (-37.5, 0)
  point P538 (-37.4401, 1.1257)
  point P539 (-37.2629, 2.2286)
  point P540 (-36.9753, 3.2871)
  point P541 (-36.5889, 4.2814)
  point P542 (-36.1187, 5.1943)
  point P543 (-35.5833, 6.0125)
  point P544 (-35.0036, 6.7266)
  point P545 (-34.4017, 7.3316)
  point P546 (-33.8006, 7.8274)
  point P547 (-33.2226, 8.2186)
  point P548 (-32.6884, 8.5142)
  point P549 (-32.2167, 8.7274)
  point P550 (-31.8227, 8.8748)
  point P551 (-31.5178, 8.9759)
  point P552 (-31.3092, 9.0521)
  point P553 (-31.1993, 9.1258)
  point P554 (-31.1859, 9.2192)
  point P555 (-31.2619, 9.3538)
  point P556 (-31.4162, 9.549)
  point P557 (-31.6335, 9.8214)
  point P558 (-31.8955, 10.1842)
  point P559 (-32.1815, 10.6463)
  point P560 (-32.4693, 11.2123)
  point P561 (-32.7362, 11.8818)
  point P562 (-32.9599, 12.6501)
  point P563 (-33.1197, 13.5076)
  point P564 (-33.1973, 14.4409)
  point P565 (-33.1775, 15.4327)
  point P566 (-33.0488, 16.4635)
  point P567 (-32.8044, 17.5112)
  point P568 (-32.4419, 18.5533)
  point P569 (-31.9636, 19.5671)
  point P570 (-31.3768, 20.5307)
  point P571 (-30.6927, 21.4244)
  point P572 (-29.9266, 22.2313)
  point P573 (-29.0971, 22.9378)
  point P574 (-28.225, 23.5347)
  point P575 (-27.3327, 24.0171)
  point P576 (-26.4429, 24.385)
  point P577 (-25.5781, 24.643)
  point P578 (-24.7591, 24.8003)
  point P579 (-24.0046, 24.8701)
  point P580 (-23.3299, 24.8693)
  point P581 (-22.7466, 24.8173)
  point P582 (-22.2618, 24.7357)
  point P583 (-21.8782, 24.647)
  point P584 (-21.5936, 24.5736)
  point P585 (-21.4011, 24.537)
  point P586 (-21.2896, 24.5567)
  point P587 (-21.2441, 24.6494)
  point P588 (-21.2464, 24.8284)
  point P589 (-21.2759, 25.1026)
  point P590 (-21.3106, 25.4767)
  point P591 (-21.328, 25.9504)
  point P592 (-21.3058, 26.5189)
  point P593 (-21.2236, 27.1727)
  point P594 (-21.0631, 27.8982)
  point P595 (-20.8092, 28.6786)
  point P596 (-20.4507, 29.4938)
  point P597 (-19.9805, 30.3222)
  point P598 (-19.3966, 31.141)
  point P599 (-18.7013, 31.9275)
  point P600 (-17.9017, 32.66)
  point P601 (-17.0094, 33.3188)
  point P602 (-16.0396, 33.8868)
  point P603 (-15.0108, 34.3506)
  point P604 (-13.9439, 34.701)
  point P605 (-12.8612, 34.9332)
  point P606 (-11.7856, 35.0471)
  point P607 (-10.7394, 35.0475)
  point P608 (-9.7436, 34.9437)
  point P609 (-8.8166, 34.7489)
  point P610 (-7.9739, 34.48)
  point P611 (-7.2269, 34.1568)
  point P612 (-6.583, 33.8009)
  point P613 (-6.0447, 33.4349)
  point P614 (-5.6098, 33.0815)
  point P615 (-5.2715, 32.7621)
  point P616 (-5.0187, 32.4965)
  point P617 (-4.8365, 32.3017)
  point P618 (-4.7067, 32.1908)
  point P619 (-4.6088, 32.1732)
  point P620 (-4.5209, 32.2535)
  point P621 (-4.4205, 32.4317)
  point P622 (-4.2855, 32.7031)
  point P623 (-4.0956, 33.0582)
  point P624 (-3.8324, 33.4838)
  point P625 (-3.4812, 33.9627)
  point P626 (-3.0306, 34.4754)
  point P627 (-2.474, 35.0001)
  point P628 (-1.809, 35.5141)
  point P629 (-1.0383, 35.9947)
  point P630 (-0.169, 36.4204)
  point P631 (0.7873, 36.7713)
  point P632 (1.8153, 37.0306)
  point P633 (2.8964, 37.1848)
  point P634 (4.0099, 37.2247)
  point P635 (5.1333, 37.1456)
  point P636 (6.2437, 36.9474)
  point P637 (7.319, 36.6349)
  point P638 (8.338, 36.2174)
  point P639 (9.2825, 35.7083)
  point P640 (10.137, 35.1245)
  point P641 (10.89, 34.4858)
  point P642 (11.5344, 33.814)
  point P643 (12.0677, 33.1316)
  point P644 (12.4922, 32.4615)
  point P645 (12.8146, 31.8252)
  point P646 (13.0461, 31.2428)
  point P647 (13.2019, 30.7311)
  point P648 (13.3001, 30.3036)
  point P649 (13.3612, 29.9697)
  point P650 (13.4072, 29.7344)
  point P651 (13.4607, 29.5976)
  point P652 (13.5437, 29.5547)
  point P653 (13.6766, 29.5968)
  point P654 (13.8777, 29.7104)
  point P655 (14.1619, 29.8788)
  point P656 (14.5402, 30.0824)
  point P657 (15.0196, 30.2996)
  point P658 (15.6021, 30.508)
  point P659 (16.2852, 30.6849)
  point P660 (17.0617, 30.8088)
  point P661 (17.9199, 30.8601)
  point P662 (18.8445, 30.8219)
  point P663 (19.817, 30.6809)
  point P664 (20.8164, 30.4279)
  point P665 (21.8203, 30.0582)
  point P666 (22.806, 29.5719)
  point P667 (23.751, 28.9737)
  point P668 (24.6346, 28.273)
  point P669 (25.4381, 27.4831)
  point P670 (26.1464, 26.6211)
  point P671 (26.748, 25.7068)
  point P672 (27.2358, 24.7617)
  point P673 (27.6073, 23.8088)
  point P674 (27.865, 22.8706)
  point P675 (28.0156, 21.9691)
  point P676 (28.0706, 21.1239)
  point P677 (28.0451, 20.3522)
  point P678 (27.9574, 19.6675)
  point P679 (27.8281, 19.0793)
  point P680 (27.6794, 18.5925)
  point P681 (27.534, 18.2073)
  point P682 (27.414, 17.9192)
  point P683 (27.34, 17.7191)
  point P684 (27.3302, 17.5941)
  point P685 (27.3998, 17.5272)
  point P686 (27.5599, 17.4993)
  point P687 (27.8174, 17.4887)
  point P688 (28.1747, 17.4731)
  point P689 (28.629, 17.4302)
  point P690 (29.1733, 17.3384)
  point P691 (29.796, 17.1783)
  point P692 (30.4818, 16.9332)
  point P693 (31.2121, 16.5898)
  point P694 (31.9661, 16.139)
  point P695 (32.7214, 15.5763)
  point P696 (33.4551, 14.9017)
  point P697 (34.145, 14.1201)
  point P698 (34.7701, 13.2409)
  point P699 (35.312, 12.2774)
  point P700 (35.7555, 11.2468)
  point P701 (36.089, 10.1688)
  point P702 (36.3057, 9.0651)
  point P703 (36.403, 7.9585)
  point P704 (36.3833, 6.8717)
  point P705 (36.2537, 5.8263)
  point P706 (36.0256, 4.8423)
  point P707 (35.7141, 3.9367)
  point P708 (35.3377, 3.123)
  point P709 (34.9171, 2.4105)
  point P710 (34.4748, 1.8043)
  point P711 (34.0333, 1.3046)
  point P712 (33.615, 0.9067)
  point P713 (33.2407, 0.6017)
  point P714 (32.9288, 0.3765)
  point P715 (32.6945, 0.2144)
  point P716 (32.5492, 0.096)
  dimension "d1" = 5
sketch "baseSketch" plane through (0, 0, 0) normal (0, 0, 1) x (1, 0, 0)
  circle A0 centre (0, 0) radius 42.5
  circle A1 centre (0, 0) radius 3
  circle A2 centre (0, 35) radius 2.5
  circle A3 centre (-16.2653, 30.991) radius 2.5
  circle A4 centre (-28.8044, 19.8823) radius 2.5
  circle A5 centre (-34.7448, 4.2188) radius 2.5
  circle A6 centre (-32.7256, -12.4112) radius 2.5
  circle A7 centre (-23.2093, -26.1979) radius 2.5
  circle A8 centre (-8.376, -33.983) radius 2.5
  circle A9 centre (8.376, -33.983) radius 2.5
  circle A10 centre (23.2093, -26.1979) radius 2.5
  circle A11 centre (32.7256, -12.4112) radius 2.5
  circle A12 centre (34.7448, 4.2188) radius 2.5
  circle A13 centre (28.8044, 19.8823) radius 2.5
  circle A14 centre (16.2653, 30.991) radius 2.5
sketch "camSketch" plane through (0, 0, 0) normal (0, 0, 1) x (1, 0, 0)
  circle A0 centre (0, 0) radius 12
  circle A1 centre (0, 3.3333) radius 3.5
extrude "Extrude1" add sketch "diskSketch" along normal blind 5 contours S2 makes body 1
extrude "Extrude2" add sketch "baseSketch" against normal blind 5 separate body contours A0 | A1 | A2 | A3 | A4 | A5 | A6 | A7 | A8 | A9 | A10 | A11 | A12 | A13 | A14 makes body 2
extrude "Extrude3" add sketch "baseSketch" along normal blind 5 separate body contours A1 makes body 3
extrude "Extrude4" add sketch "baseSketch" along normal blind 5 separate body contours A2 makes body 4
extrude "Extrude5" add sketch "baseSketch" along normal blind 5 separate body contours A3 makes body 5
extrude "Extrude6" add sketch "baseSketch" along normal blind 5 separate body contours A4 makes body 6
extrude "Extrude7" add sketch "baseSketch" along normal blind 5 separate body contours A5 makes body 7
extrude "Extrude8" add sketch "baseSketch" along normal blind 5 separate body contours A6 makes body 8
extrude "Extrude9" add sketch "baseSketch" along normal blind 5 separate body contours A7 makes body 9
extrude "Extrude10" add sketch "baseSketch" along normal blind 5 separate body contours A8 makes body 10
extrude "Extrude11" add sketch "baseSketch" along normal blind 5 separate body contours A9 makes body 11
extrude "Extrude12" add sketch "baseSketch" along normal blind 5 separate body contours A10 makes body 12
extrude "Extrude13" add sketch "baseSketch" along normal blind 5 separate body contours A11 makes body 13
extrude "Extrude14" add sketch "baseSketch" along normal blind 5 separate body contours A12 makes body 14
extrude "Extrude15" add sketch "baseSketch" along normal blind 5 separate body contours A13 makes body 15
extrude "Extrude16" add sketch "baseSketch" along normal blind 5 separate body contours A14 makes body 16
combine "Combine1" operation add target body 3 tool bodies 2 4 5 6 7 8 9 10 11 12 13 14 15 16
extrude "Extrude17" add sketch "camSketch" along normal blind 5 separate body makes body 17
equation "taperAngle1 = 0.0 deg"
named bodies: "cycloidal disk", "base", "cam"
